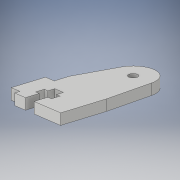
# Autodesk Inventor part: 板子8
Saved by Autodesk Inventor 2017 (Build 210142000, 142)
## iProperties
Part Number: 板子8
Material: 一般
Document SubType Name: Modeling
Designer: User
Density: 1 g/cm^3
Appearance: 預設
Author: User
Autodesk Inventor part; units mm, degrees
ref_plane "YZ Plane" through (0, 0, 0) normal (1, 0, 0) x (0, 1, 0)
ref_plane "XZ Plane" through (0, 0, 0) normal (0, 1, 0) x (-1, 0, 0)
ref_plane "XY Plane" through (0, 0, 0) normal (0, 0, 1) x (1, 0, 0)
sketch "草圖1" plane through (0, 0, 0) normal (0, 1, 0) x (-1, 0, 0)
  line L0 (12.03, 0) -> (-14.43, 0) projected
  line L1 (5.25, 0) -> (-10.4678, 0)
  line L2 (-10.65, 2.5) -> (-10.65, 16)
  line L3 (-10.65, 16) -> (5.25, 16)
  line L4 (5.25, 16) -> (5.25, 0)
  line L5 (5.25, 14.5) -> (8.25, 14.5)
  line L6 (8.25, 14.5) -> (8.25, 4.5)
  line L7 (8.25, 4.5) -> (5.25, 4.5)
  line L8 (5.25, 4.5) -> (5.25, 14.5)
  line L9 (1.5, 16) -> (-1.5, 16)
  line L10 (-1.5, 16) -> (-1.5, 12)
  line L11 (-1.5, 12) -> (1.5, 12)
  line L12 (1.5, 12) -> (1.5, 16)
  line L13 (0, -23.6) -> (0, 22.6) projected
  line L14 (2.75, 12) -> (-2.75, 12)
  line L15 (-2.75, 12) -> (-2.75, 9.5)
  line L16 (-2.75, 9.5) -> (2.75, 9.5)
  line L17 (2.75, 9.5) -> (2.75, 12)
  line L18 (1.5, 9.5) -> (-1.5, 9.5)
  line L19 (-1.5, 9.5) -> (-1.5, 7.5)
  line L20 (-1.5, 7.5) -> (1.5, 7.5)
  line L21 (1.5, 7.5) -> (1.5, 9.5)
  line L22 (-10.65, 16) -> (-3.65, 16)
  line L23 (-3.65, 16) -> (-3.65, -11)
  circle A0 centre (-3.65, -11) radius 1.3
  circle A1 centre (-3.65, -11) radius 6
  line L24 (5.25, 0) -> (2.1747, -12.4399)
  line L25 (-10.65, 16) -> (-10.65, 2.5)
  line L26 (-10.65, 2.5) -> (-9.6341, -11.4362)
  dimension "d0" = 16
  dimension "d1" = 15.9
  dimension "d2" = 3
  dimension "d3" = 10
  dimension "d4" = 1.5
  dimension "d5" = 1.5
  dimension "d6" = 3
  dimension "d7" = 4
  dimension "d8" = 2.5
  dimension "d9" = 1.25
  dimension "d10" = 1.25
  dimension "d11" = 1.5
  dimension "d12" = 3
  dimension "d13" = 2
  dimension "d14" = 9.15
  dimension "d15" = 7
  dimension "d16" = 27
  dimension "d17" = 2.6
  dimension "d18" = 12
  dimension "d19" = 13.5
  constraints: 50 end point, 10 parallel, 7 point on line, 6 perpendicular, 5 horizontal, 2 centre point, 2 coincident, 2 point on circle, 2 tangent
  measures "d0" distance of L3.end L1.start
  measures "d1" distance of L2.end L3.end
  measures "d2" distance of L6.end L7.end
  measures "d3" distance of L5.end L6.end
  measures "d4" distance between parallel lines of L3 L5
  measures "d5" distance between parallel lines of L13 L12
  measures "d6" distance of L10.end L11.end
  measures "d7" distance of L11.end L9.start
  measures "d8" distance of L16.end L14.start
  measures "d9" distance between parallel lines of L21 L17
  measures "d10" distance between parallel lines of L15 L19
  measures "d11" distance between parallel lines of L13 L21
  measures "d12" distance of L19.end L20.end
  measures "d13" distance of L18.end L19.end
  measures "d14" distance between parallel lines of L2 L10
  measures "d15" distance of L2.end L22.end
  measures "d16" distance of L22.end L23.end
  measures "d17" diameter of A0
  measures "d18" diameter of A1
  measures "d19" distance of L2.start L2.end
extrude "擠出1" add sketch "草圖1" along normal mid plane 3 contours L24 A1 L13 L0 | L0 L13 L20 L21 L16 L17 L14 L12 L3 L4 | L13 A1 L23 L0 | L0 L23 L3 L10 L14 L15 L16 L19 L20 L13 | L4 L5 L6 L7 | A1 L13 | L23 A1 L26 L0 | L0 L26 L2 L3 L23 | L13 A1
